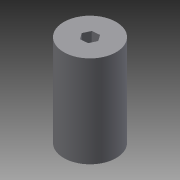
# Autodesk Inventor part: Part10
Saved by Autodesk Inventor 2015 (Build 190159000, 159)
## iProperties
Created: 2016-01-21
Part Number: Part10
Material: Generic
Document SubType Name: Modeling
Designer: 278648
Density: 1 g/cm^3
Appearance: Default
Author: 278648
Autodesk Inventor part; units mm, degrees
ref_plane "YZ Plane" through (0, 0, 0) normal (1, 0, 0) x (0, 1, 0)
ref_plane "XZ Plane" through (0, 0, 0) normal (0, 1, 0) x (-1, 0, 0)
ref_plane "XY Plane" through (0, 0, 0) normal (0, 0, 1) x (1, 0, 0)
sketch "Sketch1" plane through (0, 0, 0) normal (0, 1, 0) x (-1, 0, 0)
  circle A0 centre (0, 0) radius 25.4
  dimension "d0" = 50.8
  constraints: 1 centre point, 1 coincident
  measures "d0" diameter of A0
extrude "Extrusion1" add sketch "Sketch1" along normal blind 76.2
sketch "Sketch2" plane through (0, 76.2, 0) normal (0, 1, 0) x (1, 0, 0)
  line L0 (4.2496, -5.9753) -> (-3.0499, -6.6679)
  line L1 (-3.0499, -6.6679) -> (-7.2996, -0.6926)
  line L2 (-7.2996, -0.6926) -> (-4.2496, 5.9753)
  line L3 (-4.2496, 5.9753) -> (3.0499, 6.6679)
  line L4 (3.0499, 6.6679) -> (7.2996, 0.6926)
  line L5 (7.2996, 0.6926) -> (4.2496, -5.9753)
  point P0 (0, 0)
  point P1 (0, 0)
  dimension "d3" = 12.7
  constraints: 12 end point, 1 coincident, 13 other
  measures "d3" distance between parallel lines of L0 L3
extrude "Extrusion2" cut sketch "Sketch2" against normal through all
body "Solid1"
